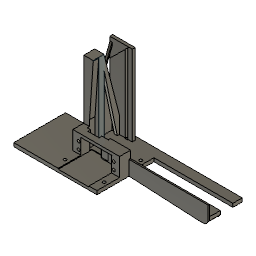
housing servo part  v2 (Autodesk Fusion 360 design; units mm, degrees)
Autodesk Fusion 360 part; units mm, degrees
note: some values were not read from the file. Chosen so that the rebuilt part matches the saved one: which face or edge a step refers to; which pieces of a blend or face edit are solid. Set by a fixed rule: which sketch regions a step uses.
sketch "Sketch1" plane through (0, 46, 0) normal (0, 1, 0) x (-1, 0, 0)
  circle A0 centre (10.45, 0) radius 2.45
  circle A1 centre (10.45, 0) radius 1.25
  line L0 (-21, 10.9962) -> (21, 10.9962)
  line L1 (21, 10.9962) -> (21, -11.1615)
  line L2 (21, -11.1615) -> (-21, -11.1615)
  line L3 (-21, -11.1615) -> (-21, 10.9962)
  line L4 (-27, 15) -> (27, 15)
  line L5 (27, 15) -> (27, -15)
  line L6 (27, -15) -> (-27, -15)
  line L7 (-27, -15) -> (-27, 15)
  constraint horizontal L0
  constraint vertical L1
  constraint horizontal L2
  constraint vertical L3
  constraint horizontal L4
  constraint vertical L5
  constraint horizontal L6
  constraint vertical L7
extrude "Extrude1" add sketch "Sketch1" against normal blind 15 contours L4 L5 L6 L7
sketch "Sketch2" plane through (0, 31, 0) normal (0, -1, 0) x (1, 0, 0)
  line L0 (21, -11.1615) -> (-21, -11.1615)
  line L1 (-21, -11.1615) -> (-21, 10.9962)
  line L2 (-21, 10.9962) -> (21, 10.9962)
  line L3 (21, 10.9962) -> (21, -11.1615)
  line L4 (-27, -15) -> (27, -15)
  line L5 (27, -15) -> (27, 15)
  line L6 (27, 15) -> (-27, 15)
  line L7 (-27, 15) -> (-27, -15)
  circle A0 centre (-24.0042, 5.0054) radius 2.4997
  line L8 (-30, 0) -> (30.3443, 0) construction
  line L9 (0, 23) -> (0, -17.7953)
  circle A1 centre (-24.0042, -5.0054) radius 2.4997
  circle A2 centre (24.0042, -5.0054) radius 2.4997
  circle A3 centre (24.0042, 5.0054) radius 2.4997
  line L10 (-27, -10) -> (-21, -10)
  line L11 (-21, -10.5) -> (21, -10.5)
  line L12 (21, -10) -> (27, -10)
  line L13 (27, -15) -> (-27, -15)
  point P0 (-24.0042, 5.0054)
  point P1 (30, 0)
  point P2 (24.0042, 5.0054)
  point P3 (-24.0042, -5.0054)
  point P4 (24.0042, 5.0054)
  point P5 (24.0042, -5.0054)
  constraint coincident P0 A0.centre
  constraint perpendicular L5 L8
  constraint perpendicular L4 L9
  constraint symmetric A0 L8 A1
  constraint symmetric A0 L9 A3
  constraint symmetric P0 L9 P4
  constraint symmetric L8.start L9 P1
  constraint symmetric L9 A1 A2
  constraint coincident P3 A1.centre
  constraint coincident P4 P2
  constraint coincident P5 A2.centre
  constraint coincident L7 L10.start
  constraint coincident L1 L10.end
  constraint perpendicular L1 L10
  constraint coincident L1 L11.start
  constraint coincident L3 L11.end
  constraint perpendicular L3 L11
  constraint coincident L3 L12.start
  constraint coincident L5 L12.end
  constraint perpendicular L5 L12
  constraint coincident L4.end L5.start
  constraint coincident L4.start L7.end
extrude "Extrude2" add sketch "Sketch2" along normal blind 31 contours L0 L3 L4 L5 L9 L12 L13 | L0 L1 L4 L7 L9 L10 L13
sketch "Sketch3" plane through (0, 46, 0) normal (0, 1, 0) x (-1, 0, 0)
  line L0 (21, -11.1615) -> (-21, -11.1615)
  line L1 (-21, -11.1615) -> (-21, 10.9962)
  line L2 (-21, 10.9962) -> (21, 10.9962)
  line L3 (21, 10.9962) -> (21, -11.1615)
  line L4 (-27, -15) -> (27, -15)
  line L5 (27, -15) -> (27, 15)
  line L6 (27, 15) -> (-27, 15)
  line L7 (-27, 15) -> (-27, -15)
  line L8 (27, -15) -> (19.1089, -15)
  line L9 (19.1089, -15) -> (19.1089, 94.6344)
  line L10 (19.1089, 94.6344) -> (27, 94.6344)
  line L11 (27, 94.6344) -> (27, -15)
  line L12 (27, -15) -> (-80, -15)
  line L13 (-80, -15) -> (-80, -10)
  line L14 (-80, -10) -> (27, -10)
  line L15 (27, -10) -> (27, -15)
  constraint horizontal L8
  constraint vertical L9
  constraint horizontal L10
  constraint vertical L11
  constraint coincident L4.end L5.start
  constraint horizontal L12
  constraint vertical L13
  constraint horizontal L14
  constraint vertical L15
extrude "Extrude3" add sketch "Sketch3" along normal blind 15 contours L0 L3 L4 L5 L8 L9 L11 L12 L14 L15 | L0 L3 L9 L14 | L0 L1 L4 L7 L9 L12 L14 | L0 L1 L9 L14 | L2 L3 L9 L14 | L2 L3 L5 L6 L9 L11 L14 | L7 L12 L13 L14 | L6 L9 L10 L11
extrude "Extrude4" add 1 faces at (27, 36, -1.6667) along direction (1, 0, 0) blind 5
extrude "Extrude5" add 1 faces at (-27, 46, -3.3333) along direction (-1, 0, 0) blind 5
sketch "Sketch4" plane through (0, 0, -10) normal (0, 0, 1) x (-1, 0, 0)
  line L0 (21, -31) -> (32, -31)
  line L1 (32, -31) -> (32, 0)
  line L2 (32, 0) -> (21, 0)
  line L3 (21, 0) -> (21, -31)
  line L4 (32, 0) -> (21, -31) construction
  line L5 (21, 0) -> (32, -31) construction
  line L6 (-32, -31) -> (-21, 0) construction
  line L7 (-32, 0) -> (-21, -31) construction
  point P0 (26.5, -15.5)
  point P1 (-26.5, -15.5)
  constraint coincident L1.end L2.start
  constraint coincident L0.start L3.end
  constraint coincident L2.end L3.start
  constraint coincident L0.end L1.start
  constraint parallel L4 L6
  constraint midpoint L5 P0
  constraint midpoint L6 P1
sketch "Sketch5" plane through (0, 61, 0) normal (0, 1, 0) x (-1, 0, 0)
  line L0 (32, 94.6344) -> (19.1089, 94.6344)
  line L1 (19.1089, 94.6344) -> (19.1089, -10)
  line L2 (19.1089, -10) -> (-80, -10)
  line L3 (-80, -10) -> (-80, -15)
  line L4 (-80, -15) -> (32, -15)
  line L5 (32, -15) -> (32, 94.6344)
  line L6 (32, -15) -> (-32, -15)
  line L7 (-32, -15) -> (-32, -10)
  line L8 (-32, -10) -> (32, -10)
  line L9 (32, -10) -> (32, -15)
  constraint horizontal L6
  constraint vertical L7
  constraint horizontal L8
  constraint vertical L9
  constraint coincident L2 L7.end
  constraint coincident L4.end L5.start
extrude "Extrude6" add sketch "Sketch5" along normal blind 10 contours L2 L4 L5 L6 L7 L8 L9
sketch "Sketch6" plane through (0, 0, -10) normal (0, 0, 1) x (-1, 0, 0)
  line L0 (-32, -46) -> (-80, -46)
  line L1 (-80, -46) -> (-80, -61)
  line L2 (-80, -61) -> (-32, -61)
  line L3 (-32, -61) -> (-32, -71)
  line L4 (-32, -71) -> (32, -71)
  line L5 (32, -71) -> (32, -61)
  line L6 (32, -61) -> (19.1089, -61)
  line L7 (19.1089, -61) -> (19.1089, -46)
  line L8 (19.1089, -46) -> (-21, -46)
  line L9 (-21, -46) -> (-32, -46)
  line L10 (-32, -61) -> (32, -61) construction
  line L11 (-32, -61) -> (-20, -71) construction
  line L12 (-20, -61) -> (-32, -71) construction
  line L13 (32, -71) -> (20, -61) construction
  line L14 (20, -71) -> (32, -61) construction
  point P0 (-26, -66)
  point P1 (26, -66)
  constraint coincident L2.end L3.start
  constraint coincident L5.end L6.start
  constraint coincident L4 L11.end
  constraint coincident L10 L12.start
  constraint coincident L3.end L4.start
  constraint coincident L4.end L5.start
  constraint coincident L6 L13.end
  constraint coincident L4 L14.start
  constraint midpoint L11 P0
  constraint midpoint L14 P1
hole "Hole1" at (-24.0042, 31, 5.0054) at (-24.0042, 31, -5.0054) at (24.0042, 31, 5.0054) at (24.0042, 31, -5.0054) direction (0, 1, 0) diameter 4 depth 5 tip angle 118
hole "Hole3" at (26, 66, -10) at (-26, 66, -10) direction (0, 0, -1) diameter 4 depth 8 tip angle 118
sketch "Sketch7" plane through (0, 0, 15) normal (0, 0, 1) x (-1, 0, 0)
  line L0 (-32, -46) -> (19.1089, -46)
  line L1 (19.1089, -46) -> (32, -46)
  line L2 (32, -46) -> (32, -31)
  line L3 (32, -31) -> (-32, -31)
  line L4 (-32, -31) -> (-32, -46)
  line L5 (19.6913, -39.1513) -> (4.3161, -39.1513)
  line L6 (4.3161, -39.1513) -> (4.3161, -46)
  line L7 (4.3161, -46) -> (19.6913, -46)
  line L8 (19.6913, -46) -> (19.6913, -39.1513)
  constraint horizontal L5
  constraint vertical L6
  constraint horizontal L7
  constraint vertical L8
  constraint coincident L0 L6.end
extrude "Extrude7" cut sketch "Sketch7" against normal blind 5 contours L0 L1 L5 L6 L7 L8
sketch "Sketch8" plane through (0, 0, -11.1615) normal (0, 0, 1) x (-1, 0, 0)
  line L0 (-21, -46) -> (21, -46)
  line L1 (21, -46) -> (21, 0)
  line L2 (21, 0) -> (-21, 0)
  line L3 (-21, 0) -> (-21, -46)
  line L4 (4.4204, -42.474) -> (-21, -42.474)
  line L5 (-21, -42.474) -> (-21, -46)
  line L6 (-21, -46) -> (4.4204, -46)
  line L7 (4.4204, -46) -> (4.4204, -42.474)
  constraint horizontal L4
  constraint vertical L5
  constraint horizontal L6
  constraint vertical L7
  constraint coincident L0.start L3.end
extrude "Extrude8" add sketch "Sketch8" along normal blind 25 contours L0 L3 L4 L5 L6 L7
sketch "Sketch10" plane through (0, 0, 0) normal (0, 0, 1) x (1, 0, 0)
  line L0 (32, 46) -> (79.9939, 46)
  line L1 (79.9939, 46) -> (79.9939, 44)
  line L2 (79.9939, 44) -> (32, 44)
  line L3 (32, 44) -> (32, 46)
  dimension "d30" = 2
  constraint horizontal L0
  constraint vertical L1
  constraint horizontal L2
  constraint vertical L3
  measures "d30" distance of L0.start L2.end
extrude "Extrude9" add sketch "Sketch10" against normal blind 15
sketch "Sketch11" plane through (0, 0, 0) normal (0, 0, 1) x (-1, 0, 0)
  line L0 (-32, -44) -> (-79.9939, -44)
  line L1 (-79.9939, -44) -> (-79.9939, -46)
  line L2 (-79.9939, -46) -> (-32, -46)
  line L3 (-32, -46) -> (-32, -44)
extrude "Extrude10" add sketch "Sketch11" along normal blind 5
sketch "Sketch12" plane through (0, 0, 94.6344) normal (0, 0, 1) x (-1, 0, 0)
  line L0 (32, -46) -> (19.1089, -46)
  line L1 (19.1089, -46) -> (19.1089, -61)
  line L2 (19.1089, -61) -> (32, -61)
  line L3 (32, -61) -> (32, -46)
  line L4 (24.1238, -53.4924) -> (-4.4206, -53.4924)
  line L5 (-4.4206, -53.4924) -> (-4.4206, -43)
  line L6 (-4.4206, -43) -> (24.1238, -43)
  line L7 (24.1238, -43) -> (24.1238, -53.4924)
  constraint horizontal L4
  constraint vertical L5
  constraint horizontal L6
  constraint vertical L7
extrude "Extrude11" cut sketch "Sketch12" against normal blind 105 contours L0 L1 L4 L7 | L0 L1 L4 L5 L6 L7
sketch "Sketch13" plane through (0, 0, 94.6344) normal (0, 0, 1) x (-1, 0, 0)
  line L0 (24.1238, -53.4924) -> (19.1089, -53.4924)
  line L1 (19.1089, -53.4924) -> (19.1089, -61)
  line L2 (19.1089, -61) -> (32, -61)
  line L3 (32, -61) -> (32, -46)
  line L4 (32, -46) -> (24.1238, -46)
  line L5 (24.1238, -46) -> (24.1238, -53.4924)
  line L6 (19.1089, -61) -> (32, -61)
  line L7 (32, -61) -> (32, -46)
  line L8 (32, -46) -> (19.1089, -46)
  line L9 (19.1089, -46) -> (19.1089, -61)
  constraint horizontal L6
  constraint vertical L7
  constraint horizontal L8
  constraint vertical L9
  constraint coincident L3.end L4.start
  constraint coincident L1.end L2.start
extrude "Extrude12" add sketch "Sketch13" along normal blind 1
draft "Draft1" angle 86 neutral plane through (-19.1089, 46, 94.6344) pull (1, 0, 0) 1 faces at (-20.7805, 48.4975, 94.6344)
sketch "Sketch17" plane through (80, 0, 0) normal (1, 0, 0) x (0, 1, 0)
  line L0 (46, -10) -> (46, -15)
  line L1 (46, -15) -> (61, -15)
  line L2 (61, -15) -> (61, -10)
  line L3 (61, -10) -> (46, -10)
  line L4 (61, -10) -> (46, -10)
  line L5 (46, -10) -> (46, -15)
  line L6 (46, -15) -> (61, -15)
  line L7 (61, -15) -> (61, -10)
  constraint horizontal L4
  constraint vertical L5
  constraint horizontal L6
  constraint vertical L7
  constraint coincident L0.end L1.start
  constraint coincident L2.end L3.start
extrude "Extrude16" add sketch "Sketch17" along normal blind 60
sketch "Sketch18" plane through (79.9939, 0, 0) normal (1, 0, 0) x (0, 1, 0)
  line L0 (44, 5) -> (44, -15)
  line L1 (44, -15) -> (46, -15)
  line L2 (46, -15) -> (46, -10)
  line L3 (46, -10) -> (46, 5)
  line L4 (46, 5) -> (44, 5)
  line L5 (44, 5) -> (46, 5)
  line L6 (46, 5) -> (46, -15)
  line L7 (46, -15) -> (44, -15)
  line L8 (44, -15) -> (44, 5)
  constraint horizontal L5
  constraint vertical L6
  constraint horizontal L7
  constraint vertical L8
  constraint coincident L1.end L2.start
  constraint coincident L0.start L4.end
extrude "Extrude17" add sketch "Sketch18" along normal blind 60
ref_plane "WorkPlane1" through (54, 35.5, -19) normal (0, 0, -1) x (1, 0, 0)
sketch "Sketch23" plane through (0, 0, -10) normal (0, 0, 1) x (-1, 0, 0)
  line L0 (-32, -31) -> (-21, -31)
  line L1 (-21, -31) -> (-21, 0)
  line L2 (-21, 0) -> (-32, 0)
  line L3 (-32, 0) -> (-32, -31)
  circle A0 centre (-27, -15) radius 2
  circle A1 centre (26.5057, -15.0373) radius 2
  dimension "d65" = 4
  dimension "d66" = 16
  dimension "d67" = 5
  dimension "d68" = 4
  measures "d65" diameter of A0
  measures "d66" distance of L0 A0.centre
  measures "d67" distance of L3 A0.centre
  measures "d68" diameter of A1
extrude "Extrude21" cut sketch "Sketch23" against normal blind 5 contours A0 | A1
sphere "SpherePrimitive1" add diameter 15 placed x (-1, 0, 0) y (0, 1, 0) z (0, 0, -1) at (133.4484, 53.3922, -19)
delete_face "DeleteFace1" 1 faces at (140.293, 50.3448, -18.6599)
sketch "Sketch20" plane through (0, 0, -15) normal (0, 0, -1) x (1, 0, 0)
  circle A0 centre (26, -66) radius 2
  circle A1 centre (-26, -66) radius 2
  line L0 (32, 0) -> (-32, 0)
  line L1 (-32, 0) -> (-32, -71)
  line L2 (-32, -71) -> (32, -71)
  line L3 (32, -71) -> (32, -61)
  line L4 (32, -61) -> (140, -61)
  line L5 (140, -61) -> (140, -46)
  line L6 (140, -46) -> (139.9939, -46)
  line L7 (139.9939, -46) -> (139.9939, -44)
  line L8 (139.9939, -44) -> (32, -44)
  line L9 (32, -44) -> (32, 0)
  line L10 (139.9091, -61) -> (129.8918, -61)
  line L11 (129.8918, -61) -> (129.8918, -44)
  line L12 (129.8918, -44) -> (139.9091, -44)
  line L13 (139.9091, -44) -> (139.9091, -61)
  circle A2 centre (27, -15) radius 2
  circle A3 centre (-26.5057, -15.0373) radius 2
  constraint horizontal L10
  constraint vertical L11
  constraint horizontal L12
  constraint vertical L13
  constraint coincident L8 L11.end
  constraint coincident L4 L10.start
extrude "Extrude18" add sketch "Sketch20" along normal blind 5 contours L4 L8 L10 L11 L12 L13
sketch "Sketch21" plane through (0, 44, 0) normal (0, -1, 0) x (1, 0, 0)
  line L0 (32, 5) -> (32, -15)
  line L1 (32, -15) -> (129.8918, -15)
  line L2 (129.8918, -15) -> (129.8918, -20)
  line L3 (129.8918, -20) -> (139.9091, -20)
  line L4 (139.9091, -20) -> (139.9091, -15)
  line L5 (139.9091, -15) -> (139.9939, -15)
  line L6 (139.9939, -15) -> (139.9939, 5)
  line L7 (139.9939, 5) -> (32, 5)
  line L8 (32, -15) -> (129.8918, -20)
  constraint coincident L0.end L1.start
  constraint coincident L2.end L3.start
extrude "Extrude19" add sketch "Sketch21" against normal blind 17 contours L1 L2 L8
fillet "Fillet1" radius 7.5 2 edges at (139.9091, 52.5, -20) (129.8918, 52.5, -20)
sketch "Sketch22" plane through (-32, 0, 0) normal (-1, 0, 0) x (0, -1, 0)
  line L0 (-71, -15) -> (0, -15)
  line L1 (0, -15) -> (0, -10)
  line L2 (0, -10) -> (-31, -10)
  line L3 (-31, -10) -> (-31, 15)
  line L4 (-31, 15) -> (-46, 15)
  line L5 (-46, 15) -> (-46, 95.6344)
  line L6 (-46, 95.6344) -> (-61, 95.6344)
  line L7 (-61, 95.6344) -> (-61, -10)
  line L8 (-61, -10) -> (-71, -10)
  line L9 (-71, -10) -> (-71, -15)
  line L10 (0, -10) -> (-71, -10)
  line L11 (-71, -10) -> (-71, -15)
  line L12 (-71, -15) -> (0, -15)
  line L13 (0, -15) -> (0, -10)
  constraint horizontal L10
  constraint vertical L11
  constraint horizontal L12
  constraint vertical L13
  constraint coincident L0.start L9.end
  constraint coincident L1.end L2.start
extrude "Extrude20" add sketch "Sketch22" along normal blind 50 contours L0 L1 L2 L8 L9 L10 L11 L12 L13
sketch "Sketch14" plane through (0, 0, -10) normal (0, 0, 1) x (-1, 0, 0)
  line L0 (21, -31) -> (32, -31)
  line L1 (32, -31) -> (32, -61)
  line L2 (82, 0) -> (21, 0)
  line L3 (21, 0) -> (21, -31)
  line L4 (26.5, -31) -> (21, -31)
  line L5 (21, -31) -> (21, -21)
  line L6 (21, -21) -> (26.5, -21)
  line L7 (26.5, -21) -> (26.5, -31)
  line L8 (-21, -31) -> (-32, -31)
  line L9 (-32, -31) -> (-32, -21)
  line L10 (-32, -21) -> (-21, -21)
  line L11 (-21, -21) -> (-21, -31)
  circle A0 centre (26.5057, -15.0373) radius 2
  line L12 (-4.4206, -53.4924) -> (-4.4206, -46)
  line L13 (-4.4206, -46) -> (-139.9939, -46)
  line L14 (-139.9939, -46) -> (-140, -46)
  line L15 (-140, -46) -> (-140, -61)
  line L16 (-140, -61) -> (-32, -61)
  line L17 (-32, -61) -> (-32, -71)
  line L18 (-32, -71) -> (82, -71)
  line L19 (82, -71) -> (82, 0)
  line L20 (32, -61) -> (19.1089, -61)
  line L21 (19.1089, -61) -> (19.1089, -53.4924)
  line L22 (19.1089, -53.4924) -> (-4.4206, -53.4924)
  circle A1 centre (-26, -66) radius 2
  circle A2 centre (26, -66) radius 2
  dimension "d43" = 10
  dimension "d44" = 10
  constraint horizontal L4
  constraint vertical L5
  constraint horizontal L6
  constraint vertical L7
  constraint coincident L3 L5.end
  constraint midpoint L0 L4.start
  constraint horizontal L8
  constraint vertical L9
  constraint horizontal L10
  constraint vertical L11
  measures "d43" distance of L8.start L10.end
  measures "d44" distance of L0.start L5.end
sketch "Sketch16" plane through (0, 0, -10) normal (0, 0, 1) x (-1, 0, 0)
  line L0 (-4.4206, -53.4924) -> (-4.4206, -46)
  line L1 (-4.4206, -46) -> (-139.9939, -46)
  line L2 (-139.9939, -46) -> (-140, -46)
  line L3 (32, -61) -> (19.1089, -61)
  line L4 (-32, -61) -> (-32, -71)
  line L5 (-32, -71) -> (82, -71)
  line L6 (32, -31) -> (32, -61)
  line L7 (19.1089, -61) -> (19.1089, -53.4924)
  line L8 (19.1089, -53.4924) -> (-4.4206, -53.4924)
  circle A0 centre (-26, -66) radius 2
  circle A1 centre (26, -66) radius 2
  line L9 (7.3442, -53.4924) -> (19.1089, -53.4924)
  line L10 (19.1089, -53.4924) -> (19.1089, -61)
  line L11 (19.1089, -61) -> (7.3442, -61)
  line L12 (7.3442, -61) -> (7.3442, -53.4924)
  line L13 (21, -31) -> (32, -31)
  line L14 (-140, -46) -> (-140, -61)
  line L15 (-140, -61) -> (-32, -61)
  line L16 (82, -71) -> (82, 0)
  line L17 (82, 0) -> (21, 0)
  line L18 (21, 0) -> (21, -31)
  circle A2 centre (26.5057, -15.0373) radius 2
  constraint horizontal L9
  constraint vertical L10
  constraint horizontal L11
  constraint vertical L12
  constraint coincident L3.end L7.start
  constraint midpoint L8 L9.start
sketch "Sketch24" plane through (0, 71, 0) normal (0, 1, 0) x (-1, 0, 0)
  line L0 (82, -10) -> (-32, -10)
  line L1 (-32, -10) -> (-32, -15)
  line L2 (-32, -15) -> (82, -15)
  line L3 (82, -15) -> (82, -10)
  line L4 (-32, -10) -> (-4.6263, -10)
  line L5 (-4.6263, -10) -> (-4.6263, -15)
  line L6 (-4.6263, -15) -> (-32, -15)
  line L7 (-32, -15) -> (-32, -10)
  constraint horizontal L4
  constraint vertical L5
  constraint horizontal L6
  constraint vertical L7
  constraint coincident L2 L5.end
  constraint coincident L0.end L1.start
extrude "Extrude22" add sketch "Sketch24" along normal blind 20 contours L0 L1 L2 L4 L5 L6 L7
sketch "Sketch25" plane through (32, 0, 0) normal (1, 0, 0) x (0, 1, 0)
  line L0 (61, -10) -> (61, -15)
  line L1 (61, -15) -> (91, -15)
  line L2 (91, -15) -> (91, -10)
  line L3 (91, -10) -> (61, -10)
sketch "Sketch26" plane through (32, 0, 0) normal (1, 0, 0) x (0, 1, 0)
  line L0 (78, -10) -> (91, -10)
  line L1 (91, -10) -> (91, -15)
  line L2 (91, -15) -> (78, -15)
  line L3 (78, -15) -> (78, -10)
  constraint horizontal L0
  constraint vertical L1
  constraint horizontal L2
  constraint vertical L3
extrude "Extrude23" add sketch "Sketch26" along normal blind 108
sketch "Sketch29" plane through (0, 61, 0) normal (0, 1, 0) x (-1, 0, 0)
  line L0 (19.1089, -10) -> (32, -10)
  line L1 (32, -10) -> (32, 95.6344)
  line L2 (32, 95.6344) -> (19.1089, 95.6344)
  line L3 (19.1089, 95.6344) -> (19.1089, -10)
  line L4 (42, 40.6344) -> (19.1089, 40.6344)
  line L5 (19.1089, 40.6344) -> (19.1089, 35.6344)
  line L6 (19.1089, 35.6344) -> (42, 35.6344)
  line L7 (42, 35.6344) -> (42, 40.6344)
  dimension "d84" = 5
  constraint horizontal L4
  constraint vertical L5
  constraint horizontal L6
  constraint vertical L7
  constraint coincident L3 L5.end
  measures "d84" distance of L4.start L6.end
sketch "Sketch30" plane through (-19.1089, 0, 0) normal (1, 0, 0) x (0, 1, 0)
  line L0 (53.4924, 94.6344) -> (53.4924, -10)
  line L1 (53.4924, -10) -> (61, -10)
  line L2 (61, -10) -> (61, 95.6344)
  line L3 (61, 95.6344) -> (46, 95.6344)
  line L4 (46, 95.6344) -> (46, 94.6344)
  line L5 (46, 94.6344) -> (53.4924, 94.6344)
sketch "Sketch33" plane through (0, 86, 0) normal (0, 1, 0) x (-1, 0, 0)
  line L0 (11.1089, 45.6344) -> (7.7089, 45.6344)
  line L1 (7.7089, 45.6344) -> (7.7089, -9.8656)
  line L2 (7.7089, -9.8656) -> (11.1089, -9.8656)
  line L3 (11.1089, -9.8656) -> (11.1089, 45.6344)
  line L4 (9.1089, 15.6344) -> (19.1089, 15.6344)
  line L5 (19.1089, -10) -> (19.1089, 95.6344)
  dimension "d95" = 3.4
  dimension "d96" = 55.5
  dimension "d114" = 8
  constraint horizontal L0
  constraint vertical L1
  constraint horizontal L2
  constraint vertical L3
  measures "d95" distance of L0.start L0.end
  measures "d96" distance of L0.start L2.end
  measures "d114" distance of L3 L5
extrude "Extrude31" add 1 faces at (4.6263, 84.3333, -11.6667) along direction (-1, 0, 0) blind 37
sketch "Sketch34" plane through (0, 0, -10) normal (0, 0, 1) x (-1, 0, 0)
  circle A0 centre (26.5057, -15.0373) radius 2
  line L0 (-4.4206, -53.4924) -> (-4.4206, -46)
  line L1 (-4.4206, -46) -> (-139.9939, -46)
  line L2 (-139.9939, -46) -> (-140, -46)
  line L3 (-140, -46) -> (-140, -61)
  line L4 (-140, -61) -> (-32, -61)
  line L5 (-32, -61) -> (-32, -78)
  line L6 (-32, -78) -> (-140, -78)
  line L7 (-140, -78) -> (-140, -91)
  line L8 (-140, -91) -> (32.3737, -91)
  line L9 (32.3737, -91) -> (32.3737, -71)
  line L10 (32.3737, -71) -> (82, -71)
  line L11 (82, -71) -> (82, 0)
  line L12 (82, 0) -> (21, 0)
  line L13 (21, 0) -> (21, -31)
  line L14 (21, -31) -> (32, -31)
  line L15 (32, -31) -> (32, -61)
  line L16 (32, -61) -> (19.1089, -61)
  line L17 (19.1089, -61) -> (19.1089, -53.4924)
  line L18 (19.1089, -53.4924) -> (-4.4206, -53.4924)
  circle A1 centre (-26, -66) radius 2
  circle A2 centre (26, -66) radius 2
  line L19 (32.3737, -81.9055) -> (1.5141, -81.9055)
  line L20 (1.5141, -81.9055) -> (1.5141, -85.9119)
  line L21 (1.5141, -85.9119) -> (32.3737, -85.9119)
  line L22 (32.3737, -85.9119) -> (32.3737, -81.9055)
  constraint horizontal L19
  constraint vertical L20
  constraint horizontal L21
  constraint vertical L22
  constraint coincident L9 L19.start
extrude "Extrude32" add sketch "Sketch34" along normal blind 60 contours L9 L19 L20 L21 L22
extrude "Extrude35" add 1 faces at (-22.0872, 84.5764, 50) along direction (0, 0, 1) blind 45
sketch "Sketch36" plane through (0, 0, -10) normal (0, 0, 1) x (-1, 0, 0)
  line L0 (1.5141, -81.9055) -> (32.3737, -81.9055)
  line L1 (32.3737, -81.9055) -> (32.3737, -71)
  line L2 (32.3737, -71) -> (82, -71)
  line L3 (82, -71) -> (82, 0)
  line L4 (82, 0) -> (21, 0)
  line L5 (21, 0) -> (21, -31)
  line L6 (21, -31) -> (32, -31)
  line L7 (32, -31) -> (32, -61)
  line L8 (32, -61) -> (19.1089, -61)
  line L9 (19.1089, -61) -> (19.1089, -53.4924)
  line L10 (19.1089, -53.4924) -> (-4.4206, -53.4924)
  line L11 (-4.4206, -53.4924) -> (-4.4206, -46)
  line L12 (-4.4206, -46) -> (-139.9939, -46)
  line L13 (-139.9939, -46) -> (-140, -46)
  line L14 (-140, -46) -> (-140, -61)
  line L15 (-140, -61) -> (-32, -61)
  line L16 (-32, -61) -> (-32, -78)
  line L17 (-32, -78) -> (-140, -78)
  line L18 (-140, -78) -> (-140, -91)
  line L19 (-140, -91) -> (32.3737, -91)
  line L20 (32.3737, -91) -> (32.3737, -85.9119)
  line L21 (32.3737, -85.9119) -> (1.5141, -85.9119)
  line L22 (1.5141, -85.9119) -> (1.5141, -81.9055)
  circle A0 centre (26.5057, -15.0373) radius 2
  circle A1 centre (-26, -66) radius 2
  circle A2 centre (26, -66) radius 2
  line L23 (29.4474, -61) -> (32.3737, -61)
  line L24 (32.3737, -61) -> (32.3737, -81.9055)
  line L25 (32.3737, -81.9055) -> (29.4474, -81.9055)
  line L26 (29.4474, -81.9055) -> (29.4474, -61)
  constraint horizontal L23
  constraint vertical L24
  constraint horizontal L25
  constraint vertical L26
  constraint coincident L0.end L1.start
  constraint coincident L8 L23.start
extrude "Extrude37" add sketch "Sketch36" along normal blind 50 contours L0 L1 L8 L23 L24 L25 L26
sketch "Sketch37" plane through (-32, 0, 0) normal (-1, 0, 0) x (0, -1, 0)
  line L0 (-61, -10) -> (-31, -10)
  line L1 (-31, -10) -> (-31, 15)
  line L2 (-31, 15) -> (-46, 15)
  line L3 (-46, 15) -> (-46, 95.6344)
  line L4 (-46, 95.6344) -> (-61, 95.6344)
  line L5 (-61, 95.6344) -> (-61, 40)
  line L6 (-61, 40) -> (-61, -10)
  line L7 (-82, 95) -> (-61, 42)
  line L8 (-61, 40) -> (-61, 42)
  line L9 (-61, 40) -> (-62, 40)
  line L10 (-62, 40) -> (-81.8505, 90.0989)
  line L11 (-82, 95) -> (-81.8505, 90.0989)
  constraint coincident L5 L7.end
  constraint coincident L5.end L6.start
  constraint perpendicular L5 L9
  constraint parallel L7 L10
extrude "Extrude38" add sketch "Sketch37" against normal blind 3 contours L5 L7 L8 L9 L10 L11
sketch "Sketch38" plane through (0, 0, 95.6344) normal (0, 0, 1) x (-1, 0, 0)
  line L0 (19.1089, -46) -> (19.1089, -61)
  line L1 (19.1089, -61) -> (32, -61)
  line L2 (32, -61) -> (32, -46)
  line L3 (32, -46) -> (19.1089, -46)
  line L4 (19.1089, -61) -> (19.1089, -85.9201)
  line L5 (11.1089, -81.4281) -> (7.7089, -81.4281)
  line L6 (7.7089, -81.4281) -> (7.7089, -86)
  line L7 (7.7089, -86) -> (11.1089, -86)
  line L8 (11.1089, -86) -> (11.1089, -81.4281)
  dimension "d115" = 3.4
  dimension "d116" = 8
  constraint coincident L0.end L1.start
  constraint perpendicular L1 L4
  constraint horizontal L5
  constraint vertical L6
  constraint horizontal L7
  constraint vertical L8
  measures "d115" distance of L5.start L5.end
  measures "d116" distance of L4 L8
extrude "Extrude39" cut sketch "Sketch38" against normal blind 106 contours L5 L6 L7 L8
sketch "Sketch39" plane through (0, 0, 95) normal (0, 0, 1) x (-1, 0, 0)
  line L0 (11.1089, -81.9055) -> (11.1089, -85.9119)
  line L1 (11.1089, -85.9119) -> (32.3737, -85.9119)
  line L2 (32.3737, -85.9119) -> (32.3737, -81.9055)
  line L3 (32.3737, -81.9055) -> (11.1089, -81.9055)
  line L4 (1.4869, -81.8712) -> (32.3737, -81.8712)
  line L5 (32.3737, -81.8712) -> (32.3737, -85.9119)
  line L6 (32.3737, -85.9119) -> (1.4869, -85.9119)
  line L7 (1.4869, -85.9119) -> (1.4869, -81.8712)
  constraint horizontal L4
  constraint vertical L5
  constraint horizontal L6
  constraint vertical L7
  constraint coincident L1.end L2.start
extrude "Extrude40" add sketch "Sketch39" along normal blind 5
draft "Draft4" angle 45 neutral plane through (-11.1089, 86, 95.6344) pull (1, 0, 0) 1 faces at (-8.8422, 83.241, 95)
sketch "Sketch40" plane through (-19.1089, 0, 0) normal (1, 0, 0) x (0, 1, 0)
  line L0 (60.9835, 75.827) -> (78.9518, -10.1031)
  line L1 (78.9518, -10.1031) -> (82.4627, -10.1031)
  line L2 (82.4627, -10.1031) -> (82.4627, 10.7607)
  line L3 (60.7242, 95.5403) -> (82.4627, 10.7607)
  line L4 (60.7242, 94.5303) -> (60.9835, 75.827)
  line L5 (60.7242, 95.5403) -> (60.7242, 94.5303)
  constraint horizontal L1
  constraint perpendicular L1 L2
  constraint vertical L5
extrude "Extrude41" add sketch "Sketch40" against normal blind 4
